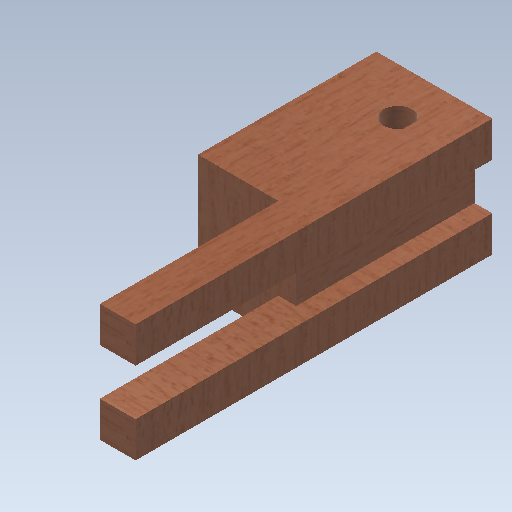
# Autodesk Inventor part: Support
Saved by Autodesk Inventor 2021.3 (Build 253353000, 353)
## iProperties
Created: 2021-06-01
Part Number: Support
Material: Wood (Oak)
Document SubType Name: Modeling
Designer: vivek
Density: 0.76 g/cm^3
Appearance: White Oak - Natural Medium Gloss
Author: vivek
Autodesk Inventor part; units mm, degrees
ref_plane "YZ Plane" through (0, 0, 0) normal (1, 0, 0) x (0, 1, 0)
ref_plane "XZ Plane" through (0, 0, 0) normal (0, 1, 0) x (-1, 0, 0)
ref_plane "XY Plane" through (0, 0, 0) normal (0, 0, 1) x (1, 0, 0)
sketch "Sketch1" plane through (0, 0, 0) normal (0, 0, 1) x (1, 0, 0)
  line L0 (27.5, -33) -> (-27.5, -33)
  line L1 (-27.5, -33) -> (-27.5, 33)
  line L2 (-27.5, 33) -> (27.5, 33)
  line L3 (27.5, 33) -> (27.5, -33)
  line L4 (0, 0) -> (0, 15.9599)
  line L5 (0, 0) -> (14.573, 0)
  point P0 (0, 33)
  point P1 (27.5, 0)
  dimension "d0" = 55
  dimension "d1" = 66
  constraints: 12 end point, 3 parallel, 2 midpoint, 2 perpendicular, 2 point on line, 1 horizontal
  measures "d0" distance of L1.end L2.end
  measures "d1" distance of L0.end L1.end
extrude "Extrusion1" add sketch "Sketch1" along normal blind 100
sketch "Sketch2" plane through (-27.5, 33, 0) normal (0, 1, 0) x (1, 0, 0)
  circle A0 centre (38, -26) radius 8 projected
  circle A1 centre (38, -26) radius 8
  point P0 (27.5, 0)
  constraints: 1 centre point, 1 coincident, 1 concentric
extrude "Extrusion2" cut sketch "Sketch2" against normal through all
sketch "Sketch3" plane through (27.5, -33, 0) normal (1, 0, 0) x (0, 0, -1)
  line L0 (0, 0) -> (-200, 0)
  line L1 (-200, 0) -> (-200, 20)
  line L2 (-200, 20) -> (0, 20)
  line L3 (0, 20) -> (0, 0)
  line L4 (0, 66) -> (-200, 66)
  line L5 (-200, 66) -> (-200, 46)
  line L6 (-200, 46) -> (0, 46)
  line L7 (0, 46) -> (0, 66)
  point P0 (0, 33)
  dimension "d6" = 200
  dimension "d7" = 20
  dimension "d8" = 200
  dimension "d9" = 20
  constraints: 16 end point, 4 parallel, 2 horizontal, 2 perpendicular
  measures "d6" distance of L1.end L2.end
  measures "d7" distance of L0.end L1.end
  measures "d8" distance of L6.end L5.end
  measures "d9" distance of L5.end L4.end
extrude "Extrusion3" add sketch "Sketch3" along normal mid plane 20
body "Solid1"
